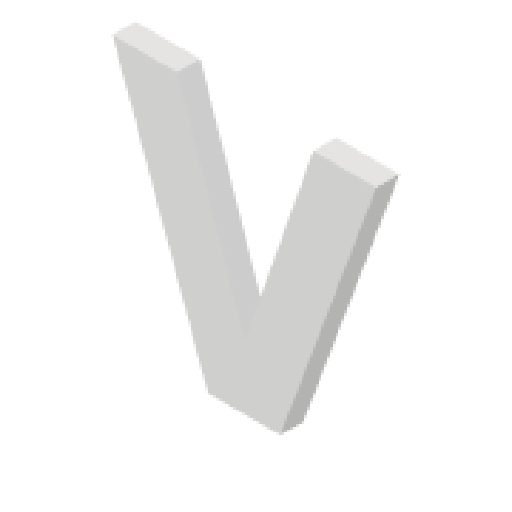
# Autodesk Inventor part: V_letter
Saved by Autodesk Inventor 2025 (Build 290162000, 162)
## iProperties
Created: 2025-01-10
Part Number: V_letter
Material: Generic
Document SubType Name: Modeling
Designer: Jan Mareš
Density: 1 g/cm^3
Appearance: Default
Author: Jan Mareš
Autodesk Inventor part; units mm, degrees
ref_plane "YZ Plane" through (0, 0, 0) normal (1, 0, 0) x (0, 1, 0)
ref_plane "XZ Plane" through (0, 0, 0) normal (0, 1, 0) x (-1, 0, 0)
ref_plane "XY Plane" through (0, 0, 0) normal (0, 0, 1) x (1, 0, 0)
sketch "Sketch1" plane through (0, 0, 0) normal (0, 0, 1) x (1, 0, 0)
  line L0 (-20, -20) -> (20, -20)
  line L1 (20, -20) -> (20, 20)
  line L2 (20, 20) -> (-20, 20)
  line L3 (-20, 20) -> (-20, -20)
  line L4 (-20, 0) -> (20, 0) construction
  line L5 (0, -28) -> (0, 28) construction
  line L6 (-28, 0) -> (28, 0) construction
  point P0 (0, 0)
  dimension "d0" = 40
  constraints: 10 end point, 3 midpoint, 2 parallel, 2 perpendicular, 1 horizontal
  measures "d0" distance of L1.end L2.end
extrude "Extrusion1" add sketch "Sketch1" along normal blind 0.6
sketch "Sketch2" plane through (0, 0, 0.6) normal (0, 0, 1) x (1, 0, 0)
  line L0 (20, -20) -> (20, 20) projected
  line L1 (20, 20) -> (-20, 20) projected
  line L2 (-20, 20) -> (-20, -20) projected
  line L3 (-20, -20) -> (20, -20) projected
  line L4 (-17.2054, 4.9978) -> (-19.7504, 12.0011) construction
  line L5 (-19.7504, 12.0011) -> (-17.859, 11.9986) construction
  line L6 (-17.859, 11.9986) -> (-16.1741, 7.0821) construction
  line L7 (-16.1741, 7.0821) -> (-14.4762, 11.9942) construction
  line L8 (-14.4762, 11.9942) -> (-12.6247, 11.9918) construction
  line L9 (-12.6247, 11.9918) -> (-15.1882, 4.9951) construction
  line L10 (-15.1882, 4.9951) -> (-17.2054, 4.9978) construction
  line L11 (-16.1745, 6.7749) -> (-17.9305, 11.8987)
  line L12 (-17.9305, 11.8987) -> (-19.6076, 11.9009)
  line L13 (-19.6076, 11.9009) -> (-17.1353, 5.0977)
  line L14 (-17.1353, 5.0977) -> (-15.2581, 5.0952)
  line L15 (-15.2581, 5.0952) -> (-12.7678, 11.8919)
  line L16 (-12.7678, 11.8919) -> (-14.405, 11.8941)
  line L17 (-14.405, 11.8941) -> (-16.1745, 6.7749)
  point P0 (0, 0)
  dimension "d3" = 0.1
  constraints: 14 end point, 6 other
  measures "d3" distance between parallel lines of L6 L11
extrude "Extrusion2" cut sketch "Sketch2" against normal up to next
body "Solid1"
